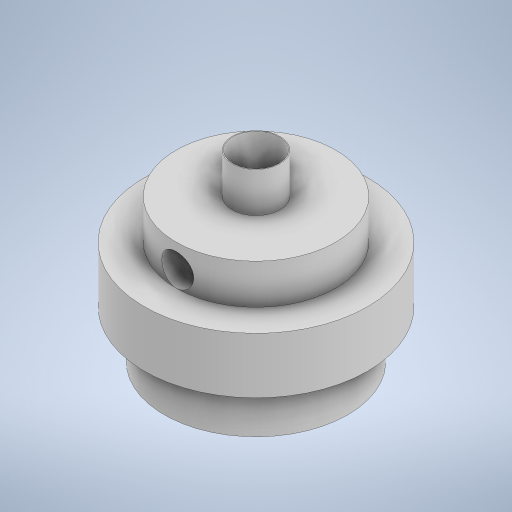
# Autodesk Inventor part: vial_adapter_male
Saved by Autodesk Inventor 2023.1 (Build 271208000, 208)
## iProperties
Created: 2023-04-28
Part Number: vial_adapter_male
Material: Generic
Document SubType Name: Modeling
Designer: dinesh
Density: 1 g/cm^3
Appearance: Default
Author: dinesh
Autodesk Inventor part; units mm, degrees
ref_plane "YZ Plane" through (0, 0, 0) normal (1, 0, 0) x (0, 1, 0)
ref_plane "XZ Plane" through (0, 0, 0) normal (0, 1, 0) x (-1, 0, 0)
ref_plane "XY Plane" through (0, 0, 0) normal (0, 0, 1) x (1, 0, 0)
sketch "Sketch1" plane through (0, 0, 0) normal (0, 0, 1) x (1, 0, 0)
  line L0 (3, 6) -> (10, 6)
  line L1 (10, 6) -> (10, 1)
  line L2 (8.5, 0) -> (2, 0)
  line L3 (2, 2) -> (2, 6)
  line L4 (0, 50) -> (0, -50)
  line L5 (2, 6) -> (3, 6) construction
  line L6 (3, 6) -> (3, 11)
  line L7 (10, 1) -> (14, 1)
  line L8 (14, 1) -> (14, 0)
  line L9 (13, 0) -> (10, 0)
  line L10 (10, 0) -> (10, 1) construction
  line L11 (14, 0) -> (13, 0) construction
  line L12 (13, 0) -> (13, -6)
  line L13 (13, -6) -> (14, -6)
  line L14 (14, -6) -> (14, 0)
  line L15 (11.5, 0) -> (10.5, 0)
  arc A0 (2, 2) -> (4, 0) centre (4, 2) ccw
  line L16 (-4.5, 0) -> (4.5, 0) construction
  line L17 (10.5, 0) -> (11.5, 0)
  line L18 (11.5, 0) -> (11.5, -6)
  line L19 (11.5, -6) -> (10.5, -6) construction
  line L20 (10.5, -6) -> (10.5, -6)
  arc A1 (10.5, -6) -> (4.5, 0) centre (4.5, -6) ccw
  line L21 (3, 11) -> (2.9, 11)
  line L22 (2.9, 11) -> (2, 6)
  line L23 (11.5, -6) -> (11.5, -12)
  line L24 (11.5, -12) -> (11.4, -12)
  line L25 (11.4, -12) -> (10.5, -6)
  point P0 (0, 0)
  point P1 (4.5, 0)
  dimension "d0" = 4
  dimension "d1" = 6
  dimension "d2" = 20
  dimension "d5" = 1
  dimension "d6" = 26
  dimension "d7" = 1
  dimension "d8" = 6
  dimension "d11" = 5
  dimension "d12" = 100
  dimension "d15" = 1
  dimension "d16" = 1.5
  dimension "d17" = 15
  dimension "d26" = 0.1
  dimension "d27" = 1
  dimension "d28" = 5
  dimension "d29" = 6
  dimension "d30" = 0.1
  constraints: 52 end point, 8 horizontal, 8 parallel, 6 perpendicular, 4 midpoint, 4 point on circle, 4 tangent, 3 collinear, 3 point on line, 2 centre point, 2 vertical
  measures "d0" diameter of L3 L4
  measures "d1" distance between parallel lines of L0 L2
  measures "d2" diameter of L1 L4
  measures "d5" distance between parallel lines of L9 L7
  measures "d6" diameter of L12 L4
  measures "d7" distance between parallel lines of L12 L14
  measures "d8" distance between parallel lines of L13 L9
  measures "d12" distance of L4.start L4.end
  measures "d15" distance between parallel lines of L18 L20
  measures "d16" distance between parallel lines of L12 L18
  measures "d26" distance of L6.end L21.end
  measures "d27" distance between parallel lines of L3 L6
  measures "d28" distance of L0.start L6.end
  measures "d29" distance of L18.end L23.end
  measures "d30" distance of L23.end L24.end
revolve "Revolution1" add sketch "Sketch1" angle 360 about axis through (0, 50, 0) along (0, -1, 0)
sketch "Sketch2" plane through (0, 0, 0) normal (0, 0, 1) x (1, 0, 0)
  line L0 (-2, 11) -> (2, 11) projected
  line L1 (-2, 2) -> (2, 2) construction
  line L2 (-3, 11) -> (3, 11) projected
  line L3 (0, 11) -> (0, 2) construction
  line L4 (-3, 6) -> (3, 6) projected
  circle A0 centre (0, 3) radius 2
  line L5 (-4, 0) -> (4, 0) projected
  point P0 (0, 0)
  point P1 (1.7321, 2)
  point P2 (-1.7321, 2)
  dimension "d19" = 4
  dimension "d25" = 3
  constraints: 2 end point, 2 midpoint, 1 centre point, 1 point on line
  measures "d19" diameter of A0
  measures "d25" distance from line of L5 A0.centre
extrude "Extrusion1" cut sketch "Sketch2" along normal blind 20 and the other way blind 2.1
equation "\"d0\" = t_D"
equation "\"d1\" = top_th + w_th"
equation "\"d2\" = top_D"
equation "\"d5\" = w_th"
equation "\"d6\" = lv_OD"
equation "\"d7\" = w_th"
equation "\"d8\" = w_l"
equation "\"d11\" = fillet_D"
equation "\"d15\" = w_th"
equation "\"d16\" = lv_th"
equation "\"d17\" = 3 * fillet_D"
equation "\"d26\" = tol"
equation "\"d27\" = w_th"
equation "\"d28\" = cn_h"
equation "\"d29\" = w_l"
equation "\"d30\" = tol"
equation "\"d19\" = t_D"
equation "\"d25\" = 0.5 * t_D + w_th"
equation "\"d21\" = top_D"
equation "\"d22\" = 0.5 * t_D + tol"
equation "\"tol\" = 0.1"
equation "\"fillet_D\" = 5"
equation "\"w_th\" = 1"
equation "\"w_l\" = 6"
equation "\"t_D\" = 4"
equation "\"top_D\" = 20"
equation "\"top_th\" = t_D + w_th"
equation "\"cn_h\" = 5"
equation "\"lv_OD\" = 26"
equation "\"lv_thickness\" = 1.5"
equation "\"sv_OD\" = 13"
equation "\"sv_thickness\" = 1.5"
equation "\"sv_th\" = 1.5"
equation "\"lv_th\" = 1.5"
equation "\"t_D_f\" = t_D + 2 * w_th"
equation "\"top_th_f\" = t_D_f + cn_h"
equation "\"hw_length\" = 6"
equation "\"ft_D\" = 4"
equation "\"hw_thickness\" = 1"
body "Solid1"
